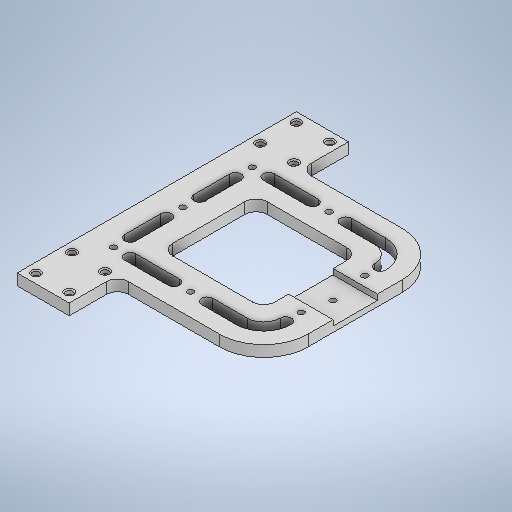
# Autodesk Inventor part: Chassis Rear Spine 2
Saved by Autodesk Inventor 2025.2 (Build 292293000, 293)
## iProperties
Created: 2025-02-20
Part Number: Chassis Rear Spine 2
Material: Generic
Document SubType Name: Modeling
Designer: Matt Tidd
Density: 1 g/cm^3
Appearance: Default
Author: Matt Tidd
Autodesk Inventor part; units mm, degrees
ref_plane "YZ Plane" through (0, 0, 0) normal (1, 0, 0) x (0, 1, 0)
ref_plane "XZ Plane" through (0, 0, 0) normal (0, 1, 0) x (-1, 0, 0)
ref_plane "XY Plane" through (0, 0, 0) normal (0, 0, 1) x (1, 0, 0)
sketch "Sketch1" plane through (0, 0, 0) normal (0, 1, 0) x (-1, 0, 0)
  line L0 (-23.5, 126) -> (23.5, 126)
  line L1 (23.5, 126) -> (23.5, -126)
  line L2 (23.5, -126) -> (-23.5, -126)
  line L3 (-23.5, -126) -> (-23.5, 126)
  line L4 (-23.5, 22.5) -> (-23.5, 62.5)
  line L5 (23.5, 0) -> (-23.5, 0) construction
  line L6 (-23.5, -82.5) -> (-23.5, -42.5)
  line L7 (-23.5, 82.5) -> (-23.5, 42.5)
  line L8 (-23.5, -42.5) -> (-115.5, -42.5)
  line L9 (-115.5, -42.5) -> (-115.5, -82.5)
  line L10 (-115.5, -82.5) -> (-23.5, -82.5)
  line L11 (-23.5, -82.5) -> (-23.5, -42.5)
  line L12 (-23.5, 42.5) -> (-115.5, 42.5)
  line L13 (-115.5, 42.5) -> (-115.5, 82.5)
  line L14 (-115.5, 82.5) -> (-23.5, 82.5)
  line L15 (-23.5, 82.5) -> (-23.5, 42.5)
  arc A0 (-155.5, -42.5) -> (-115.5, -82.5) centre (-115.5, -42.5) ccw
  arc A1 (-115.5, 82.5) -> (-155.5, 42.5) centre (-115.5, 42.5) ccw
  line L16 (-115.5, -42.5) -> (-155.5, -42.5)
  line L17 (-155.5, -42.5) -> (-155.5, 42.5)
  line L18 (-155.5, 42.5) -> (-115.5, 42.5)
  line L19 (-115.5, 42.5) -> (-115.5, -42.5)
  circle A2 centre (15, -117.5) radius 1.8
  circle A3 centre (-15, -117.5) radius 1.8
  circle A4 centre (15, -85) radius 1.8
  circle A5 centre (-15, -85) radius 1.8
  circle A6 centre (15, 117.5) radius 1.8
  circle A7 centre (-15, 117.5) radius 1.8
  circle A8 centre (15, 85) radius 1.8
  circle A9 centre (-15, 85) radius 1.8
  point P0 (0, 0)
  point P1 (-23.5, -62.5)
  dimension "d0" = 47
  dimension "d1" = 252
  dimension "d8" = 92
  dimension "d9" = 40
  dimension "d10" = 92
  dimension "d11" = 40
  dimension "d12" = 3.6
  dimension "d13" = 3.6
  dimension "d14" = 3.6
  dimension "d15" = 3.6
  constraints: 40 end point, 10 centre point, 8 parallel, 5 symmetric about line, 4 horizontal, 4 perpendicular, 4 point on circle, 3 point on line, 2 coincident, 2 midpoint, 4 other
  measures "d0" distance of L1.end L2.end
  measures "d1" distance of L0.end L1.end
  measures "d8" distance of L10.end L9.end
  measures "d9" distance of L9.end L8.end
  measures "d10" distance of L13.end L14.end
  measures "d11" distance of L12.end L13.end
  measures "d12" diameter of A2
  measures "d13" diameter of A3
  measures "d14" diameter of A4
  measures "d15" diameter of A5
extrude "Extrusion1" add sketch "Sketch1" along normal blind 10 contours L0 L1 L2 L3 | L3 L12 L13 L14 | L13 L18 A1 | L19 L16 L17 L18 | L10 L9 L8 L3 | L9 A0 L16
sketch "Sketch2" plane through (0, 10, 0) normal (0, 1, 0) x (1, 0, 0)
  circle A0 centre (15, 117.5) radius 1.8 projected
  circle A1 centre (15, 117.5) radius 3.25
  circle A2 centre (15, 85) radius 1.8 projected
  circle A3 centre (15, 85) radius 3.25
  circle A4 centre (-15, 85) radius 1.8 projected
  circle A5 centre (-15, 85) radius 3.25
  circle A6 centre (-15, 117.5) radius 1.8 projected
  circle A7 centre (-15, 117.5) radius 3.25
  circle A8 centre (15, -85) radius 1.8 projected
  circle A9 centre (15, -85) radius 3.25
  circle A10 centre (-15, -85) radius 1.8 projected
  circle A11 centre (-15, -85) radius 3.25
  circle A12 centre (-15, -117.5) radius 1.8 projected
  circle A13 centre (-15, -117.5) radius 3.25
  circle A14 centre (15, -117.5) radius 1.8 projected
  circle A15 centre (15, -117.5) radius 3.25
  point P0 (0, 0)
  dimension "d18" = 6.5
  dimension "d19" = 6.5
  dimension "d20" = 6.5
  dimension "d21" = 6.5
  dimension "d22" = 6.5
  dimension "d23" = 6.5
  dimension "d24" = 6.5
  dimension "d25" = 6.5
  constraints: 8 centre point, 8 coincident
  measures "d18" diameter of A1
  measures "d19" diameter of A3
  measures "d20" diameter of A5
  measures "d21" diameter of A7
  measures "d22" diameter of A9
  measures "d23" diameter of A11
  measures "d24" diameter of A13
  measures "d25" diameter of A15
extrude "Extrusion2" cut sketch "Sketch2" against normal blind 4 contours A0 | A1 | A3 | A5 | A7 | A9 | A11 | A13 | A15
fillet "Fillet1" radius 1 8 edges at (-18.25, 10, -117.5) (11.75, 10, -117.5) (-18.25, 10, -85) (11.75, 10, -85) (-18.25, 10, 85) (11.75, 10, 85) (11.75, 10, 117.5) (-18.25, 10, 117.5)
sketch "Sketch3" plane through (155.5, 0, 42.5) normal (1, 0, 0) x (0, 0, -1)
  line L0 (85, 10) -> (0, 10) construction
  line L1 (0, 0) -> (85, 0) projected
  line L2 (22.5, 10) -> (62.5, 10)
  line L3 (62.5, 10) -> (62.5, 5)
  line L4 (62.5, 5) -> (22.5, 5)
  line L5 (22.5, 5) -> (22.5, 10)
  point P0 (42.5, 0)
  dimension "d33" = 40
  dimension "d34" = 5
  constraints: 8 end point, 2 parallel, 1 horizontal, 1 perpendicular, 1 point on line
  measures "d33" distance of L3.end L4.end
  measures "d34" distance of L2.end L3.end
extrude "Extrusion3" cut sketch "Sketch3" against normal blind 40
sketch "Sketch4" plane through (0, 10, 0) normal (0, 1, 0) x (1, 0, 0)
  line L0 (-23.5, 126) -> (-23.5, -126) construction
  line L1 (-23.5, 0) -> (155.5, 0) construction
  line L2 (155.5, -42.5) -> (155.5, 42.5) construction
  line L3 (135.5, -82.5) -> (135.5, 82.5) construction
  line L4 (0, -82.5) -> (0, 82.5) construction
  line L5 (-23.5, 62.5) -> (155.5, 62.5) construction
  line L6 (-23.5, -62.5) -> (155.5, -62.5) construction
  circle A0 centre (0, 0) radius 2.75
  circle A1 centre (69.5, -62.5) radius 2.75
  circle A2 centre (135.5, 0) radius 2.75
  circle A3 centre (69.5, 62.5) radius 2.75
  circle A4 centre (0, 62.5) radius 2.75
  circle A5 centre (0, -62.5) radius 2.75
  dimension "d35" = 5.5
  dimension "d36" = 5.5
  dimension "d37" = 5.5
  dimension "d38" = 5.5
  dimension "d39" = 5.5
  dimension "d40" = 5.5
  constraints: 10 end point, 6 centre point, 5 coincident, 5 point on line, 4 midpoint, 3 symmetric about line, 2 vertical, 1 perpendicular
  measures "d35" diameter of A0
  measures "d36" diameter of A1
  measures "d37" diameter of A2
  measures "d38" diameter of A3
  measures "d39" diameter of A4
  measures "d40" diameter of A5
extrude "Extrusion4" cut sketch "Sketch4" against normal through all
fillet "Fillet2" radius 10 6 edges at (23.5, 5, -42.5) (115.5, 5, -42.5) (23.5, 5, 42.5) (115.5, 5, 42.5) (23.5, 5, -82.5) (23.5, 5, 82.5)
sketch "Sketch5" plane through (0, 10, 0) normal (0, 1, 0) x (1, 0, 0)
  line L0 (-23.5, 126) -> (-23.5, -126) construction
  line L1 (-23.5, 0) -> (155.5, 0) construction
  line L2 (155.5, -42.5) -> (155.5, 42.5) construction
  arc A0 (155.5, 42.5) -> (115.5, 82.5) centre (115.5, 42.5) ccw construction
  line L3 (115.5, 82.5) -> (115.5, 42.5) construction
  line L4 (115.5, 42.5) -> (155.5, 42.5) construction
  line L5 (155.5, -42.5) -> (115.5, -42.5) construction
  arc A1 (115.5, -82.5) -> (155.5, -42.5) centre (115.5, -42.5) ccw construction
  line L6 (115.5, -42.5) -> (115.5, -82.5) construction
  line L7 (135.5, -35) -> (135.5, -62.5) construction
  line L8 (135.5, -62.5) -> (84.5, -62.5) construction
  line L9 (135.5, 35) -> (135.5, 62.5) construction
  line L10 (135.5, 62.5) -> (84.5, 62.5) construction
  arc A2 (135.5, 42.5) -> (115.5, 62.5) centre (115.5, 42.5) ccw construction
  arc A3 (140.5, 42.5) -> (115.5, 67.5) centre (115.5, 42.5) ccw
  arc A4 (130.5, 42.5) -> (115.5, 57.5) centre (115.5, 42.5) ccw
  arc A5 (130.5, 42.5) -> (140.5, 42.5) centre (135.5, 42.5) ccw
  arc A6 (115.5, 67.5) -> (115.5, 57.5) centre (115.5, 62.5) ccw
  arc A7 (115.5, -62.5) -> (135.5, -42.5) centre (115.5, -42.5) ccw construction
  arc A8 (115.5, -67.5) -> (140.5, -42.5) centre (115.5, -42.5) ccw
  arc A9 (115.5, -57.5) -> (130.5, -42.5) centre (115.5, -42.5) ccw
  arc A10 (115.5, -57.5) -> (115.5, -67.5) centre (115.5, -62.5) ccw
  arc A11 (140.5, -42.5) -> (130.5, -42.5) centre (135.5, -42.5) ccw
  line L11 (84.5, -62.5) -> (115.5, -62.5) construction
  line L12 (84.5, -67.5) -> (115.5, -67.5)
  line L13 (115.5, -57.5) -> (84.5, -57.5)
  arc A12 (84.5, -57.5) -> (84.5, -67.5) centre (84.5, -62.5) ccw
  arc A13 (115.5, -67.5) -> (115.5, -57.5) centre (115.5, -62.5) ccw
  line L14 (84.5, 62.5) -> (115.5, 62.5) construction
  line L15 (84.5, 57.5) -> (115.5, 57.5)
  line L16 (115.5, 67.5) -> (84.5, 67.5)
  arc A14 (84.5, 67.5) -> (84.5, 57.5) centre (84.5, 62.5) ccw
  arc A15 (115.5, 57.5) -> (115.5, 67.5) centre (115.5, 62.5) ccw
  line L17 (15, 62.5) -> (54.5, 62.5) construction
  line L18 (15, 57.5) -> (54.5, 57.5)
  line L19 (54.5, 67.5) -> (15, 67.5)
  arc A16 (15, 67.5) -> (15, 57.5) centre (15, 62.5) ccw
  arc A17 (54.5, 57.5) -> (54.5, 67.5) centre (54.5, 62.5) ccw
  line L20 (15, -62.5) -> (54.5, -62.5) construction
  line L21 (15, -67.5) -> (54.5, -67.5)
  line L22 (54.5, -57.5) -> (15, -57.5)
  arc A18 (15, -57.5) -> (15, -67.5) centre (15, -62.5) ccw
  arc A19 (54.5, -67.5) -> (54.5, -57.5) centre (54.5, -62.5) ccw
  line L23 (0, -15) -> (0, -47.5) construction
  line L24 (-5, -15) -> (-5, -47.5)
  line L25 (5, -47.5) -> (5, -15)
  arc A20 (5, -15) -> (-5, -15) centre (0, -15) ccw
  arc A21 (-5, -47.5) -> (5, -47.5) centre (0, -47.5) ccw
  line L26 (0, 15) -> (0, 47.5) construction
  line L27 (23.5, -32.5) -> (23.5, 32.5) projected
  line L28 (5, 15) -> (5, 47.5)
  line L29 (-5, 47.5) -> (-5, 15)
  arc A22 (-5, 15) -> (5, 15) centre (0, 15) ccw
  arc A23 (5, 47.5) -> (-5, 47.5) centre (0, 47.5) ccw
  point P0 (0, 0)
  point P1 (100, -62.5)
  point P2 (100, 62.5)
  point P3 (34.75, 62.5)
  point P4 (34.75, -62.5)
  point P5 (0, -31.25)
  point P6 (0, 31.25)
  dimension "d44" = 10
  dimension "d45" = 10
  dimension "d46" = 10
  dimension "d47" = 10
  dimension "d48" = 10
  dimension "d49" = 10
  constraints: 66 end point, 44 point on circle, 33 tangent, 22 centre point, 10 midpoint, 9 parallel, 6 perpendicular, 4 symmetric about line, 3 vertical, 2 coincident, 2 point on line, 1 collinear, 1 horizontal
  measures "d44" diameter of A6
  measures "d45" diameter of A11
  measures "d46" diameter of A17
  measures "d47" diameter of A19
  measures "d48" diameter of A21
  measures "d49" diameter of A23
extrude "Extrusion5" cut sketch "Sketch5" against normal blind 10
sketch "Sketch6" plane through (0, 10, 0) normal (0, 1, 0) x (1, 0, 0)
  point P0 (0, 0)
  point P1 (0, 85)
sketch "Sketch7" plane through (0, 10, 0) normal (0, 1, 0) x (1, 0, 0)
  circle A0 centre (135.5, 28.75) radius 2.75
  line L0 (115.5, 32.5) -> (115.5, -32.5) construction
  line L1 (115.5, 0) -> (155.5, 0) construction
  line L2 (155.5, -42.5) -> (155.5, 42.5) construction
  circle A1 centre (135.5, -28.75) radius 2.75
  point P0 (0, 0)
  dimension "d52" = 5.5
  dimension "d53" = 5.5
  constraints: 2 centre point, 2 end point, 2 midpoint
  measures "d52" diameter of A0
  measures "d53" diameter of A1
extrude "Extrusion6" cut sketch "Sketch7" against normal blind 10
equation "\"d50\" = d48"
equation "\"d54\" = d48"
body "Solid1"
